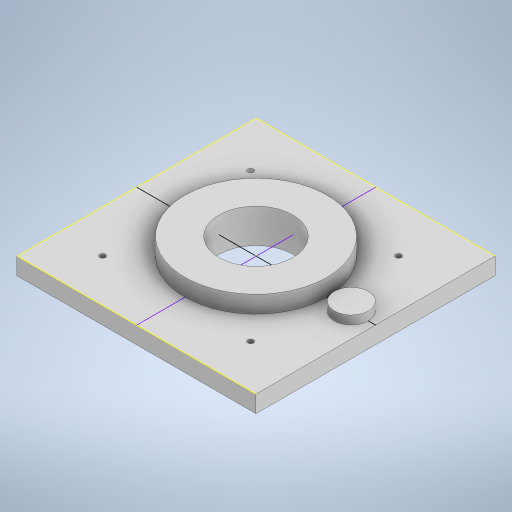
# Autodesk Inventor part: fan_num1
Saved by Autodesk Inventor 2024 (Build 280153000, 153)
## iProperties
Created: 2024-08-06
Part Number: fan_num1
Material: 일반
Document SubType Name: Modeling
Designer: chlqj
Density: 1 g/cm^3
Appearance: 기본값
Author: chlqj
Autodesk Inventor part; units mm, degrees
ref_plane "YZ Plane" through (0, 0, 0) normal (1, 0, 0) x (0, 1, 0)
ref_plane "XZ Plane" through (0, 0, 0) normal (0, 1, 0) x (-1, 0, 0)
ref_plane "XY Plane" through (0, 0, 0) normal (0, 0, 1) x (1, 0, 0)
sketch "스케치9" plane through (0, 0, 0) normal (0, 1, 0) x (-1, 0, 0)
  line L0 (21, 21) -> (-21, 21)
  line L1 (-21, 21) -> (-21, -21)
  line L2 (-21, -21) -> (21, -21)
  line L3 (21, -21) -> (21, 21)
  line L4 (21, 21) -> (-21, -21)
  line L5 (21, -21) -> (-21, 21)
  point P0 (0, 0)
  point P1 (0, 0)
  dimension "d25" = 42
  dimension "d26" = 42
  constraints: 12 end point, 2 parallel, 1 coincident, 1 horizontal, 1 midpoint, 1 perpendicular
  measures "d25" distance of L2.end L0.start
  measures "d26" distance of L1.end L2.end
extrude "돌출3" add sketch "스케치9" along normal blind 3
sketch "스케치10" plane through (0, 3, 0) normal (0, 1, 0) x (1, 0, 0)
  point P0 (0, 0)
hole "구멍1" at (0, 3, 0) direction (0, -1, 0) diameter 13 end through all
sketch "스케치11" plane through (0, 3, 0) normal (0, 1, 0) x (1, 0, 0)
  circle A0 centre (0, 0) radius 12.5
  circle A1 centre (0, 0) radius 6.5
  dimension "d36" = 25
  constraints: 2 centre point, 2 coincident
  measures "d36" diameter of A0
extrude "돌출4" add sketch "스케치11" along normal blind 3
sketch "스케치12" plane through (0, 3, 0) normal (0, 1, 0) x (1, 0, 0)
  line L0 (-21, 21) -> (-21, -21) projected
  line L1 (21, 21) -> (-21, 21) projected
  line L2 (-21, -21) -> (21, -21) projected
  line L3 (0, -21) -> (0, 21)
  line L4 (-21, 0) -> (21, 0)
  point P0 (0, 0)
  constraints: 4 end point, 2 midpoint, 1 horizontal
sketch "스케치13" plane through (0, 3, 0) normal (0, 1, 0) x (1, 0, 0)
  line L0 (-13.4728, -13.4728) -> (12.5272, -13.4728)
  line L1 (12.5272, -13.4728) -> (12.5272, 12.5272)
  line L2 (12.5272, 12.5272) -> (-13.4728, 12.5272)
  line L3 (-13.4728, 12.5272) -> (-13.4728, -13.4728)
  point P0 (0, 0)
  dimension "d41" = 26
  dimension "d42" = 26
  constraints: 8 end point, 2 parallel, 1 horizontal, 1 perpendicular
  measures "d41" distance of L2.end L0.start
  measures "d42" distance of L0.start L0.end
hole "구멍2" at (-13.4728, 3, 13.4728) at (-13.4728, 3, -12.5272) at (12.5272, 3, -12.5272) at (12.5272, 3, 13.4728) direction (0, -1, 0) diameter 1 end through all
sketch "스케치14" plane through (0, 3, 0) normal (0, 1, 0) x (1, 0, 0)
  line L0 (21, 21) -> (-21, 21) projected
  line L1 (0, 21) -> (21, 0)
  line L2 (21, -21) -> (21, 21) projected
  line L3 (21, 0) -> (0.0421, -20.9579)
  line L4 (21, 0) -> (12.5, 0)
  circle A0 centre (0, 0) radius 12.5 projected
  circle A1 centre (16.75, 0) radius 3.0052
  constraints: 6 end point, 3 midpoint, 1 centre point, 1 horizontal, 1 horizontal alignment, 1 tangent, 1 other
extrude "돌출5" add sketch "스케치14" along normal blind 1.5 contours A1 L4 | A1 L4
